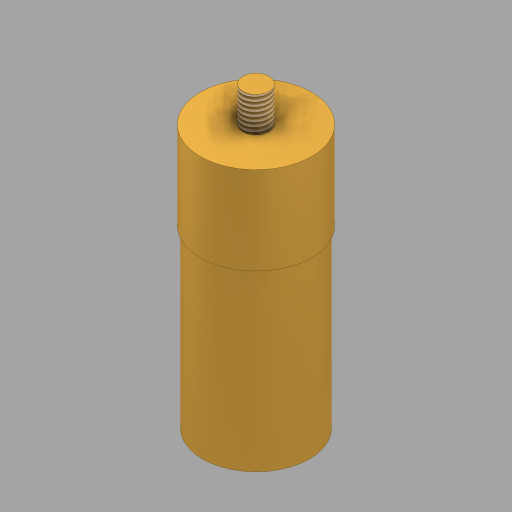
# Autodesk Inventor part: tubeFitting
Saved by Autodesk Inventor 2024 (Build 280153020, 153B)
## iProperties
Created: 2023-10-26
Part Number: tubeFitting
Material: Brass, Soft Yellow
Document SubType Name: Modeling
Designer: schanen
Density: 8.47 g/cm^3
Appearance: Brass - Satin
Mass: 21.161 g
Surface Area: 11.0937 cm^2
Volume: 2.49835 cm^3
Author: schanen
Autodesk Inventor part; units mm, degrees
ref_plane "YZ Plane" through (0, 0, 0) normal (1, 0, 0) x (0, 1, 0)
ref_plane "XZ Plane" through (0, 0, 0) normal (0, 1, 0) x (-1, 0, 0)
ref_plane "XY Plane" through (0, 0, 0) normal (0, 0, 1) x (1, 0, 0)
sketch "Sketch1" plane through (0, 0, 0) normal (0, 0, 1) x (1, 0, 0)
  line L0 (0, 34) -> (-1.5, 34)
  line L1 (-1.5, 34) -> (-1.5, 30)
  line L2 (-1.5, 30) -> (-6.35, 30)
  line L3 (-6.35, 30) -> (-6.35, 20)
  line L4 (-6.35, 20) -> (-6.096, 20)
  line L5 (-6.096, 20) -> (-6.096, 0)
  line L6 (-6.096, 0) -> (0, 0)
  line L7 (0, 0) -> (0, 34)
  dimension "d0" = 1.5
  dimension "d2" = 6.096
  dimension "d3" = 20
  dimension "d4" = 4
  dimension "d5" = 10
  dimension "d9" = 6.35
  constraints: 16 end point, 7 perpendicular, 1 coincident, 1 horizontal
  measures "d0" distance between parallel lines of L7 L1
  measures "d2" distance between parallel lines of L7 L5
  measures "d3" distance of L4.end L5.end
  measures "d4" distance of L0.end L1.end
  measures "d5" distance of L2.end L3.end
  measures "d9" distance between parallel lines of L7 L3
revolve "Revolution1" add sketch "Sketch1" angle 360 about axis through (0, 0, 0) along (0, 1, 0)
thread "Thread1" size "M3x0.5" class "6g" standard "ANSI Metric M Profile" full length
equation "\"d2\" = 0.5 * tube_od - tube_wall"
equation "\"d9\" = 0.5 * tube_od"
equation "\"tube_od\" = 12.7"
equation "\"tube_wall\" = 0.254"
body "Solid1"
